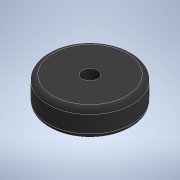
# Autodesk Inventor part: Wheels
Saved by Autodesk Inventor 2022 (Build 260153000, 153)
## iProperties
Created: 2021-11-05
Part Number: Wheels
Material: Generic
Document SubType Name: Modeling
Designer: Mark Maara
Density: 1 g/cm^3
Appearance: Rubber - Black
Author: Mark Maara
Autodesk Inventor part; units mm, degrees
ref_plane "YZ Plane" through (0, 0, 0) normal (1, 0, 0) x (0, 1, 0)
ref_plane "XZ Plane" through (0, 0, 0) normal (0, 1, 0) x (-1, 0, 0)
ref_plane "XY Plane" through (0, 0, 0) normal (0, 0, 1) x (1, 0, 0)
sketch "Sketch1" plane through (0, 0, 0) normal (0, 1, 0) x (-1, 0, 0)
  circle A0 centre (0, 0) radius 125
  circle A1 centre (0, 0) radius 22.5
  dimension "d0" = 250
  dimension "d6" = 45
  constraints: 2 centre point, 2 coincident
  measures "d0" diameter of A0
  measures "d6" diameter of A1
extrude "Extrusion1" add sketch "Sketch1" along normal blind 80
fillet "Fillet1" radius 15 2 edges at (125, 80, 0) (125, 0, 0)
body "Solid1"
